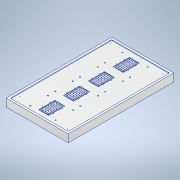
# Autodesk Inventor part: Tamale Assembly Plate 0p625in
Saved by Autodesk Inventor 2022 (Build 260153000, 153)
## iProperties
Created: 2021-07-29
Part Number: Tamale Assembly Plate 0p625in
Material: Aluminum 6061
Document SubType Name: Modeling
Designer: Caleb
Density: 2.7 g/cm^3
Appearance: Aluminum - Flat
Author: Caleb
Autodesk Inventor part; units mm, degrees
ref_plane "YZ Plane" through (0, 0, 0) normal (1, 0, 0) x (0, 1, 0)
ref_plane "XZ Plane" through (0, 0, 0) normal (0, 1, 0) x (-1, 0, 0)
ref_plane "XY Plane" through (0, 0, 0) normal (0, 0, 1) x (1, 0, 0)
sketch "Sketch1" plane through (0, 0, 0) normal (0, 1, 0) x (-1, 0, 0)
  line L0 (-63.5, -107.95) -> (63.5, -107.95)
  line L1 (63.5, -107.95) -> (63.5, 107.95)
  line L2 (63.5, 107.95) -> (-63.5, 107.95)
  line L3 (-63.5, 107.95) -> (-63.5, -107.95)
  line L4 (-63.5, -107.95) -> (63.5, 107.95) construction
  line L5 (63.5, -107.95) -> (-63.5, 107.95) construction
  point P0 (0, 0)
  dimension "d0" = 127
  dimension "d1" = 215.9
  constraints: 12 end point, 2 midpoint, 2 parallel, 1 horizontal, 1 perpendicular
  measures "d0" distance of L2.end L1.end
  measures "d1" distance of L0.end L1.end
extrude "Extrusion1" add sketch "Sketch1" along normal blind 15.875
sketch "Sketch2" plane through (0, 15.875, 0) normal (0, 1, 0) x (1, 0, 0)
  line L0 (57.15, 103.6) -> (-57.15, 103.6)
  line L1 (-59.15, 101.6) -> (-59.15, -101.6)
  line L2 (-57.15, -103.6) -> (57.15, -103.6)
  line L3 (59.15, -101.6) -> (59.15, 101.6)
  line L4 (59.15, 103.6) -> (-59.15, -103.6) construction
  line L5 (-59.15, 103.6) -> (59.15, -103.6) construction
  line L6 (-63.5, -107.95) -> (63.5, -107.95) projected
  line L7 (-63.5, 107.95) -> (-63.5, -107.95) projected
  line L8 (63.5, 107.95) -> (-63.5, 107.95) projected
  line L9 (63.5, -107.95) -> (63.5, 107.95) projected
  arc A0 (-59.15, -101.6) -> (-57.15, -103.6) centre (-57.15, -101.6) ccw
  arc A1 (57.15, -103.6) -> (59.15, -101.6) centre (57.15, -101.6) ccw
  arc A2 (59.15, 101.6) -> (57.15, 103.6) centre (57.15, 101.6) ccw
  arc A3 (-57.15, 103.6) -> (-59.15, 101.6) centre (-57.15, 101.6) ccw
  point P0 (0, 0)
  dimension "d4" = 4.35
  dimension "d5" = 4.35
  dimension "d6" = 4.35
  dimension "d77" = 2
  constraints: 12 end point, 8 point on circle, 8 point on line, 8 tangent, 4 centre point, 3 equal radius, 2 midpoint, 2 parallel, 1 horizontal, 1 perpendicular
  measures "d4" distance between parallel lines of L2 L6
  measures "d5" distance between parallel lines of L0 L8
  measures "d6" distance between parallel lines of L7 L1
  measures "d77" radius of A0
extrude "Extrusion2" cut sketch "Sketch2" against normal blind 1.6 contours A2 L3 A1 L2 A0 L1 A3 L0
sketch "Sketch3" plane through (0, 14.275, 0) normal (0, 1, 0) x (1, 0, 0)
  line L0 (-59.15, -101.6) -> (-59.15, 101.6) projected
  line L1 (57.15, -103.6) -> (-57.15, -103.6) projected
  point P0 (0, 0)
  point P1 (-26.75, -95.25)
  point P2 (-26.75, -59.15)
  point P3 (24.75, -95.25)
  point P4 (24.75, -59.15)
  point P5 (-57.15, -101.6)
  point P6 (-57.15, 101.6)
  point P7 (57.15, -101.6)
  point P8 (-26.75, -44.45)
  point P9 (24.75, -44.45)
  point P10 (24.75, -8.35)
  point P11 (-26.75, -8.35)
  point P12 (-26.75, 6.35)
  point P13 (24.75, 6.35)
  point P14 (24.75, 42.45)
  point P15 (-26.75, 42.45)
  point P16 (-26.75, 57.15)
  point P17 (24.75, 57.15)
  point P18 (24.75, 93.25)
  point P19 (-26.75, 93.25)
  point P20 (-59.15, 101.6)
  point P21 (-57.15, -103.6)
  dimension "d9" = 32.4
  dimension "d10" = 8.35
  dimension "d11" = 36.1
  dimension "d12" = 51.5
  dimension "d15" = 50.8
  constraints: 14 vertical alignment, 2 horizontal alignment, 2 other
  measures "d11" distance of point (-26.75, -59.15) point (-26.75, -95.25)
  measures "d12" distance of point (24.75, -59.15) point (-26.75, -59.15)
  measures "d15" distance of point (-26.75, -95.25) point (-26.75, -44.45)
hole "Hole1" at (-26.75, 14.275, 95.25) at (-26.75, 14.275, 59.15) at (24.75, 14.275, 95.25) at (24.75, 14.275, 59.15) at (-26.75, 14.275, 44.45) at (24.75, 14.275, 44.45) at (24.75, 14.275, 8.35) at (-26.75, 14.275, 8.35) at (-26.75, 14.275, -6.35) at (24.75, 14.275, -6.35) at (24.75, 14.275, -42.45) at (-26.75, 14.275, -42.45) at (-26.75, 14.275, -57.15) at (24.75, 14.275, -57.15) at (24.75, 14.275, -93.25) at (-26.75, 14.275, -93.25) direction (0, -1, 0) diameter 2.5 end through all
sketch "Sketch4" plane through (0, 14.275, 0) normal (0, 1, 0) x (1, 0, 0)
  line L0 (-59.15, -101.6) -> (-59.15, 101.6) projected
  line L1 (57.15, -103.6) -> (-57.15, -103.6) projected
  line L2 (59.15, 101.6) -> (59.15, -101.6) projected
  line L3 (-57.15, 103.6) -> (57.15, 103.6) projected
  point P0 (0, 0)
  point P1 (-54.15, -88.9)
  point P2 (-57.15, -101.6)
  point P3 (-57.15, 101.6)
  point P4 (57.15, -101.6)
  point P5 (52.155, -98.61)
  point P6 (52.155, 96.6)
  point P7 (-54.135, 96.6)
  point P8 (57.15, 101.6)
  point P9 (-12.765, -85.2)
  point P10 (-12.765, -69.2)
  point P11 (10.766, -85.2)
  point P12 (10.766, -69.2)
  point P13 (-12.765, -34.4)
  point P14 (-12.765, -18.4)
  point P15 (10.766, -18.4)
  point P16 (10.766, -34.4)
  point P17 (-12.765, 16.4)
  point P18 (-12.765, 32.4)
  point P19 (10.766, 32.4)
  point P20 (10.766, 16.4)
  point P21 (-12.765, 67.2)
  point P22 (-12.765, 83.2)
  point P23 (10.766, 83.2)
  point P24 (10.766, 67.2)
  point P25 (-59.15, 101.6)
  point P26 (-57.15, -103.6)
  point P27 (59.15, -101.6)
  point P28 (57.15, 103.6)
  dimension "d35" = 46.385
  dimension "d36" = 18.4
  dimension "d37" = 16
  dimension "d38" = 23.531
  dimension "d41" = 50.8
  dimension "d98" = 3.7
  dimension "d99" = 41.385
  dimension "d100" = 13.41
  dimension "d101" = 64.92
  dimension "d102" = 181.8
  dimension "d103" = 41.37
  dimension "d104" = 181.8
  dimension "d105" = 64.92
  constraints: 14 vertical alignment, 2 horizontal alignment, 4 other
  measures "d37" distance of point (-12.765, -69.2) point (-12.765, -85.2)
  measures "d38" distance of point (10.766, -85.2) point (-12.765, -85.2)
  measures "d41" distance of point (-12.765, -85.2) point (-12.765, -34.4)
  measures "d98" vertical distance of point (-54.15, -88.9) point (-12.765, -85.2)
  measures "d99" horizontal distance of point (-12.765, -85.2) point (-54.15, -88.9)
  measures "d100" vertical distance of point (52.155, -98.61) point (-12.765, -85.2)
  measures "d101" horizontal distance of point (52.155, -98.61) point (-12.765, -85.2)
  measures "d102" vertical distance of point (-12.765, -85.2) point (-54.135, 96.6)
  measures "d103" horizontal distance of point (-12.765, -85.2) point (-54.135, 96.6)
  measures "d104" vertical distance of point (52.155, 96.6) point (-12.765, -85.2)
  measures "d105" horizontal distance of point (52.155, 96.6) point (-12.765, -85.2)
hole "Hole2" at (-54.15, 14.275, 88.9) at (52.155, 14.275, 98.61) at (52.155, 14.275, -96.6) at (-54.135, 14.275, -96.6) at (-12.765, 14.275, 85.2) at (-12.765, 14.275, 69.2) at (10.766, 14.275, 85.2) at (10.766, 14.275, 69.2) at (-12.765, 14.275, 34.4) at (-12.765, 14.275, 18.4) at (10.766, 14.275, 18.4) at (10.766, 14.275, 34.4) at (-12.765, 14.275, -16.4) at (-12.765, 14.275, -32.4) at (10.766, 14.275, -32.4) at (10.766, 14.275, -16.4) at (-12.765, 14.275, -67.2) at (-12.765, 14.275, -83.2) at (10.766, 14.275, -83.2) at (10.766, 14.275, -67.2) direction (0, -1, 0) diameter 1.0211 end through all thread size "00-96 NS" class "2B" standard "ANSI Unified Screw Threads"
sketch "Sketch5" plane through (0, 14.275, 0) normal (0, 1, 0) x (1, 0, 0)
  line L0 (57.15, -103.6) -> (-57.15, -103.6) projected
  line L1 (-59.15, -101.6) -> (-59.15, 101.6) projected
  point P0 (0, 0)
  point P1 (-7.35, -89.9)
  point P2 (57.15, -101.6)
  point P3 (-57.15, -101.6)
  point P4 (-57.15, 101.6)
  point P5 (-7.35, -86.725)
  point P6 (-7.35, -83.55)
  point P7 (-7.35, -80.375)
  point P8 (-7.35, -77.2)
  point P9 (-7.35, -74.025)
  point P10 (-7.35, -70.85)
  point P11 (-7.35, -67.675)
  point P12 (-7.35, -64.5)
  point P13 (-4.175, -89.9)
  point P14 (-4.175, -86.725)
  point P15 (-4.175, -83.55)
  point P16 (-4.175, -80.375)
  point P17 (-4.175, -77.2)
  point P18 (-4.175, -74.025)
  point P19 (-4.175, -70.85)
  point P20 (-4.175, -67.675)
  point P21 (-4.175, -64.5)
  point P22 (-1, -89.9)
  point P23 (-1, -86.725)
  point P24 (-1, -83.55)
  point P25 (-1, -80.375)
  point P26 (-1, -77.2)
  point P27 (-1, -74.025)
  point P28 (-1, -70.85)
  point P29 (-1, -67.675)
  point P30 (-1, -64.5)
  point P31 (2.175, -89.9)
  point P32 (2.175, -86.725)
  point P33 (2.175, -83.55)
  point P34 (2.175, -80.375)
  point P35 (2.175, -77.2)
  point P36 (2.175, -74.025)
  point P37 (2.175, -70.85)
  point P38 (2.175, -67.675)
  point P39 (2.175, -64.5)
  point P40 (5.35, -89.9)
  point P41 (5.35, -86.725)
  point P42 (5.35, -83.55)
  point P43 (5.35, -80.375)
  point P44 (5.35, -77.2)
  point P45 (5.35, -74.025)
  point P46 (5.35, -70.85)
  point P47 (5.35, -67.675)
  point P48 (5.35, -64.5)
  point P49 (5.35, -13.7)
  point P50 (5.35, -16.875)
  point P51 (5.35, -20.05)
  point P52 (5.35, -23.225)
  point P53 (5.35, -26.4)
  point P54 (5.35, -29.575)
  point P55 (5.35, -32.75)
  point P56 (5.35, -35.925)
  point P57 (5.35, -39.1)
  point P58 (2.175, -13.7)
  point P59 (2.175, -16.875)
  point P60 (2.175, -20.05)
  point P61 (2.175, -23.225)
  point P62 (2.175, -26.4)
  point P63 (2.175, -29.575)
  point P64 (2.175, -32.75)
  point P65 (2.175, -35.925)
  point P66 (2.175, -39.1)
  point P67 (-1, -13.7)
  point P68 (-1, -16.875)
  point P69 (-1, -20.05)
  point P70 (-1, -23.225)
  point P71 (-1, -26.4)
  point P72 (-1, -29.575)
  point P73 (-1, -32.75)
  point P74 (-1, -35.925)
  point P75 (-1, -39.1)
  point P76 (-4.175, -13.7)
  point P77 (-4.175, -16.875)
  point P78 (-4.175, -20.05)
  point P79 (-4.175, -23.225)
  point P80 (-4.175, -26.4)
  point P81 (-4.175, -29.575)
  point P82 (-4.175, -32.75)
  point P83 (-4.175, -35.925)
  point P84 (-4.175, -39.1)
  point P85 (-7.35, -13.7)
  point P86 (-7.35, -16.875)
  point P87 (-7.35, -20.05)
  point P88 (-7.35, -23.225)
  point P89 (-7.35, -26.4)
  point P90 (-7.35, -29.575)
  point P91 (-7.35, -32.75)
  point P92 (-7.35, -35.925)
  point P93 (-7.35, -39.1)
  point P94 (5.35, 37.1)
  point P95 (5.35, 33.925)
  point P96 (5.35, 30.75)
  point P97 (5.35, 27.575)
  point P98 (5.35, 24.4)
  point P99 (5.35, 21.225)
  point P100 (5.35, 18.05)
  point P101 (5.35, 14.875)
  point P102 (5.35, 11.7)
  point P103 (2.175, 37.1)
  point P104 (2.175, 33.925)
  point P105 (2.175, 30.75)
  point P106 (2.175, 27.575)
  point P107 (2.175, 24.4)
  point P108 (2.175, 21.225)
  point P109 (2.175, 18.05)
  point P110 (2.175, 14.875)
  point P111 (2.175, 11.7)
  point P112 (-1, 37.1)
  point P113 (-1, 33.925)
  point P114 (-1, 30.75)
  point P115 (-1, 27.575)
  point P116 (-1, 24.4)
  point P117 (-1, 21.225)
  point P118 (-1, 18.05)
  point P119 (-1, 14.875)
  point P120 (-1, 11.7)
  point P121 (-4.175, 37.1)
  point P122 (-4.175, 33.925)
  point P123 (-4.175, 30.75)
  point P124 (-4.175, 27.575)
  point P125 (-4.175, 24.4)
  point P126 (-4.175, 21.225)
  point P127 (-4.175, 18.05)
  point P128 (-4.175, 14.875)
  point P129 (-4.175, 11.7)
  point P130 (-7.35, 37.1)
  point P131 (-7.35, 33.925)
  point P132 (-7.35, 30.75)
  point P133 (-7.35, 27.575)
  point P134 (-7.35, 24.4)
  point P135 (-7.35, 21.225)
  point P136 (-7.35, 18.05)
  point P137 (-7.35, 14.875)
  point P138 (-7.35, 11.7)
  point P139 (5.35, 87.9)
  point P140 (5.35, 84.725)
  point P141 (5.35, 81.55)
  point P142 (5.35, 78.375)
  point P143 (5.35, 75.2)
  point P144 (5.35, 72.025)
  point P145 (5.35, 68.85)
  point P146 (5.35, 65.675)
  point P147 (5.35, 62.5)
  point P148 (2.175, 87.9)
  point P149 (2.175, 84.725)
  point P150 (2.175, 81.55)
  point P151 (2.175, 78.375)
  point P152 (2.175, 75.2)
  point P153 (2.175, 72.025)
  point P154 (2.175, 68.85)
  point P155 (2.175, 65.675)
  point P156 (2.175, 62.5)
  point P157 (-1, 87.9)
  point P158 (-1, 84.725)
  point P159 (-1, 81.55)
  point P160 (-1, 78.375)
  point P161 (-1, 75.2)
  point P162 (-1, 72.025)
  point P163 (-1, 68.85)
  point P164 (-1, 65.675)
  point P165 (-1, 62.5)
  point P166 (-4.175, 87.9)
  point P167 (-4.175, 84.725)
  point P168 (-4.175, 81.55)
  point P169 (-4.175, 78.375)
  point P170 (-4.175, 75.2)
  point P171 (-4.175, 72.025)
  point P172 (-4.175, 68.85)
  point P173 (-4.175, 65.675)
  point P174 (-4.175, 62.5)
  point P175 (-7.35, 87.9)
  point P176 (-7.35, 84.725)
  point P177 (-7.35, 81.55)
  point P178 (-7.35, 78.375)
  point P179 (-7.35, 75.2)
  point P180 (-7.35, 72.025)
  point P181 (-7.35, 68.85)
  point P182 (-7.35, 65.675)
  point P183 (-7.35, 62.5)
  point P184 (-57.15, -103.6)
  point P185 (-59.15, 101.6)
  dimension "d53" = 13.7
  dimension "d54" = 51.8
  dimension "d57" = 3.175
  dimension "d60" = 3.175
  dimension "d65" = 50.8
  constraints: 143 vertical alignment, 36 horizontal alignment, 2 other
  measures "d57" distance of point (-7.35, -89.9) point (-7.35, -86.725)
  measures "d60" distance of point (-7.35, -89.9) point (-4.175, -89.9)
  measures "d65" distance of point (5.35, -64.5) point (5.35, -13.7)
hole "Hole3" at (-7.35, 14.275, 89.9) at (-7.35, 14.275, 86.725) at (-7.35, 14.275, 83.55) at (-7.35, 14.275, 80.375) at (-7.35, 14.275, 77.2) at (-7.35, 14.275, 74.025) at (-7.35, 14.275, 70.85) at (-7.35, 14.275, 67.675) at (-7.35, 14.275, 64.5) at (-4.175, 14.275, 89.9) at (-4.175, 14.275, 86.725) at (-4.175, 14.275, 83.55) at (-4.175, 14.275, 80.375) at (-4.175, 14.275, 77.2) at (-4.175, 14.275, 74.025) at (-4.175, 14.275, 70.85) at (-4.175, 14.275, 67.675) at (-4.175, 14.275, 64.5) at (-1, 14.275, 89.9) at (-1, 14.275, 86.725) at (-1, 14.275, 83.55) at (-1, 14.275, 80.375) at (-1, 14.275, 77.2) at (-1, 14.275, 74.025) at (-1, 14.275, 70.85) at (-1, 14.275, 67.675) at (-1, 14.275, 64.5) at (2.175, 14.275, 89.9) at (2.175, 14.275, 86.725) at (2.175, 14.275, 83.55) at (2.175, 14.275, 80.375) at (2.175, 14.275, 77.2) at (2.175, 14.275, 74.025) at (2.175, 14.275, 70.85) at (2.175, 14.275, 67.675) at (2.175, 14.275, 64.5) at (5.35, 14.275, 89.9) at (5.35, 14.275, 86.725) at (5.35, 14.275, 83.55) at (5.35, 14.275, 80.375) at (5.35, 14.275, 77.2) at (5.35, 14.275, 74.025) at (5.35, 14.275, 70.85) at (5.35, 14.275, 67.675) at (5.35, 14.275, 64.5) at (5.35, 14.275, 13.7) at (5.35, 14.275, 16.875) at (5.35, 14.275, 20.05) at (5.35, 14.275, 23.225) at (5.35, 14.275, 26.4) direction (0, -1, 0) diameter 1.6 end through all and at (5.35, 14.275, 29.575) (5.35, 14.275, 32.75) (5.35, 14.275, 35.925) (5.35, 14.275, 39.1) (2.175, 14.275, 13.7) (2.175, 14.275, 16.875) (2.175, 14.275, 20.05) (2.175, 14.275, 23.225) (2.175, 14.275, 26.4) (2.175, 14.275, 29.575) (2.175, 14.275, 32.75) (2.175, 14.275, 35.925) (2.175, 14.275, 39.1) (-1, 14.275, 13.7) (-1, 14.275, 16.875) (-1, 14.275, 20.05) (-1, 14.275, 23.225) (-1, 14.275, 26.4) (-1, 14.275, 29.575) (-1, 14.275, 32.75) (-1, 14.275, 35.925) (-1, 14.275, 39.1) (-4.175, 14.275, 13.7) (-4.175, 14.275, 16.875) (-4.175, 14.275, 20.05) (-4.175, 14.275, 23.225) (-4.175, 14.275, 26.4) (-4.175, 14.275, 29.575) (-4.175, 14.275, 32.75) (-4.175, 14.275, 35.925) (-4.175, 14.275, 39.1) (-7.35, 14.275, 13.7) (-7.35, 14.275, 16.875) (-7.35, 14.275, 20.05) (-7.35, 14.275, 23.225) (-7.35, 14.275, 26.4) (-7.35, 14.275, 29.575) (-7.35, 14.275, 32.75) (-7.35, 14.275, 35.925) (-7.35, 14.275, 39.1) (5.35, 14.275, -37.1) (5.35, 14.275, -33.925) (5.35, 14.275, -30.75) (5.35, 14.275, -27.575) (5.35, 14.275, -24.4) (5.35, 14.275, -21.225) (5.35, 14.275, -18.05) (5.35, 14.275, -14.875) (5.35, 14.275, -11.7) (2.175, 14.275, -37.1) (2.175, 14.275, -33.925) (2.175, 14.275, -30.75) (2.175, 14.275, -27.575) (2.175, 14.275, -24.4) (2.175, 14.275, -21.225) (2.175, 14.275, -18.05) (2.175, 14.275, -14.875) (2.175, 14.275, -11.7) (-1, 14.275, -37.1) (-1, 14.275, -33.925) (-1, 14.275, -30.75) (-1, 14.275, -27.575) (-1, 14.275, -24.4) (-1, 14.275, -21.225) (-1, 14.275, -18.05) (-1, 14.275, -14.875) (-1, 14.275, -11.7) (-4.175, 14.275, -37.1) (-4.175, 14.275, -33.925) (-4.175, 14.275, -30.75) (-4.175, 14.275, -27.575) (-4.175, 14.275, -24.4) (-4.175, 14.275, -21.225) (-4.175, 14.275, -18.05) (-4.175, 14.275, -14.875) (-4.175, 14.275, -11.7) (-7.35, 14.275, -37.1) (-7.35, 14.275, -33.925) (-7.35, 14.275, -30.75) (-7.35, 14.275, -27.575) (-7.35, 14.275, -24.4) (-7.35, 14.275, -21.225) (-7.35, 14.275, -18.05) (-7.35, 14.275, -14.875) (-7.35, 14.275, -11.7) (5.35, 14.275, -87.9) (5.35, 14.275, -84.725) (5.35, 14.275, -81.55) (5.35, 14.275, -78.375) (5.35, 14.275, -75.2) (5.35, 14.275, -72.025) (5.35, 14.275, -68.85) (5.35, 14.275, -65.675) (5.35, 14.275, -62.5) (2.175, 14.275, -87.9) (2.175, 14.275, -84.725) (2.175, 14.275, -81.55) (2.175, 14.275, -78.375) (2.175, 14.275, -75.2) (2.175, 14.275, -72.025) (2.175, 14.275, -68.85) (2.175, 14.275, -65.675) (2.175, 14.275, -62.5) (-1, 14.275, -87.9) (-1, 14.275, -84.725) (-1, 14.275, -81.55) (-1, 14.275, -78.375) (-1, 14.275, -75.2) (-1, 14.275, -72.025) (-1, 14.275, -68.85) (-1, 14.275, -65.675) (-1, 14.275, -62.5) (-4.175, 14.275, -87.9) (-4.175, 14.275, -84.725) (-4.175, 14.275, -81.55) (-4.175, 14.275, -78.375) (-4.175, 14.275, -75.2) (-4.175, 14.275, -72.025) (-4.175, 14.275, -68.85) (-4.175, 14.275, -65.675) (-4.175, 14.275, -62.5) (-7.35, 14.275, -87.9) (-7.35, 14.275, -84.725) (-7.35, 14.275, -81.55) (-7.35, 14.275, -78.375) (-7.35, 14.275, -75.2) (-7.35, 14.275, -72.025) (-7.35, 14.275, -68.85) (-7.35, 14.275, -65.675) (-7.35, 14.275, -62.5)
sketch "Sketch6" plane through (0, 14.275, 0) normal (0, 1, 0) x (1, 0, 0)
  line L0 (5.95, -62.4) -> (-7.95, -62.4)
  line L1 (-9.45, -63.9) -> (-9.45, -90.5)
  line L2 (-7.95, -92) -> (5.95, -92)
  line L3 (7.45, -90.5) -> (7.45, -63.9)
  line L4 (7.982, -60.368) -> (-9.982, -60.368)
  line L5 (-11.482, -61.868) -> (-11.482, -92.532)
  line L6 (-9.982, -94.032) -> (7.982, -94.032)
  line L7 (9.482, -92.532) -> (9.482, -61.868)
  circle A0 centre (-7.35, -64.5) radius 0.8 projected
  circle A1 centre (-7.35, -89.9) radius 0.8 projected
  circle A2 centre (5.35, -89.9) radius 0.8 projected
  arc A3 (-9.45, -90.5) -> (-7.95, -92) centre (-7.95, -90.5) ccw
  arc A4 (-11.482, -92.532) -> (-9.982, -94.032) centre (-9.982, -92.532) ccw
  arc A5 (-9.982, -60.368) -> (-11.482, -61.868) centre (-9.982, -61.868) ccw
  arc A6 (-7.95, -62.4) -> (-9.45, -63.9) centre (-7.95, -63.9) ccw
  arc A7 (7.45, -63.9) -> (5.95, -62.4) centre (5.95, -63.9) ccw
  arc A8 (9.482, -61.868) -> (7.982, -60.368) centre (7.982, -61.868) ccw
  arc A9 (7.982, -94.032) -> (9.482, -92.532) centre (7.982, -92.532) ccw
  arc A10 (5.95, -92) -> (7.45, -90.5) centre (5.95, -90.5) ccw
  line L8 (-7.95, -41.2) -> (5.95, -41.2)
  line L9 (-9.982, -43.232) -> (7.982, -43.232)
  arc A11 (5.95, -41.2) -> (7.45, -39.7) centre (5.95, -39.7) ccw
  arc A12 (7.982, -43.232) -> (9.482, -41.732) centre (7.982, -41.732) ccw
  arc A13 (-9.45, -39.7) -> (-7.95, -41.2) centre (-7.95, -39.7) ccw
  arc A14 (-11.482, -41.732) -> (-9.982, -43.232) centre (-9.982, -41.732) ccw
  line L10 (5.95, -11.6) -> (-7.95, -11.6)
  line L11 (-9.45, -13.1) -> (-9.45, -39.7)
  line L12 (7.45, -39.7) -> (7.45, -13.1)
  line L13 (7.982, -9.568) -> (-9.982, -9.568)
  line L14 (-11.482, -11.068) -> (-11.482, -41.732)
  line L15 (9.482, -41.732) -> (9.482, -11.068)
  arc A15 (-7.95, -11.6) -> (-9.45, -13.1) centre (-7.95, -13.1) ccw
  arc A16 (-9.982, -9.568) -> (-11.482, -11.068) centre (-9.982, -11.068) ccw
  arc A17 (9.482, -11.068) -> (7.982, -9.568) centre (7.982, -11.068) ccw
  arc A18 (7.45, -13.1) -> (5.95, -11.6) centre (5.95, -13.1) ccw
  line L16 (-7.95, 9.6) -> (5.95, 9.6)
  line L17 (-9.982, 7.568) -> (7.982, 7.568)
  arc A19 (5.95, 9.6) -> (7.45, 11.1) centre (5.95, 11.1) ccw
  arc A20 (7.982, 7.568) -> (9.482, 9.068) centre (7.982, 9.068) ccw
  arc A21 (-9.45, 11.1) -> (-7.95, 9.6) centre (-7.95, 11.1) ccw
  arc A22 (-11.482, 9.068) -> (-9.982, 7.568) centre (-9.982, 9.068) ccw
  line L18 (5.95, 39.2) -> (-7.95, 39.2)
  line L19 (-9.45, 37.7) -> (-9.45, 11.1)
  line L20 (7.45, 11.1) -> (7.45, 37.7)
  line L21 (7.982, 41.232) -> (-9.982, 41.232)
  line L22 (-11.482, 39.732) -> (-11.482, 9.068)
  line L23 (9.482, 9.068) -> (9.482, 39.732)
  arc A23 (-7.95, 39.2) -> (-9.45, 37.7) centre (-7.95, 37.7) ccw
  arc A24 (-9.982, 41.232) -> (-11.482, 39.732) centre (-9.982, 39.732) ccw
  arc A25 (9.482, 39.732) -> (7.982, 41.232) centre (7.982, 39.732) ccw
  arc A26 (7.45, 37.7) -> (5.95, 39.2) centre (5.95, 37.7) ccw
  line L24 (-7.95, 60.4) -> (5.95, 60.4)
  line L25 (-9.982, 58.368) -> (7.982, 58.368)
  arc A27 (5.95, 60.4) -> (7.45, 61.9) centre (5.95, 61.9) ccw
  arc A28 (7.982, 58.368) -> (9.482, 59.868) centre (7.982, 59.868) ccw
  arc A29 (-9.45, 61.9) -> (-7.95, 60.4) centre (-7.95, 61.9) ccw
  arc A30 (-11.482, 59.868) -> (-9.982, 58.368) centre (-9.982, 59.868) ccw
  line L26 (5.95, 90) -> (-7.95, 90)
  line L27 (-9.45, 88.5) -> (-9.45, 61.9)
  line L28 (7.45, 61.9) -> (7.45, 88.5)
  line L29 (7.982, 92.032) -> (-9.982, 92.032)
  line L30 (-11.482, 90.532) -> (-11.482, 59.868)
  line L31 (9.482, 59.868) -> (9.482, 90.532)
  arc A31 (-7.95, 90) -> (-9.45, 88.5) centre (-7.95, 88.5) ccw
  arc A32 (-9.982, 92.032) -> (-11.482, 90.532) centre (-9.982, 90.532) ccw
  arc A33 (9.482, 90.532) -> (7.982, 92.032) centre (7.982, 90.532) ccw
  arc A34 (7.45, 88.5) -> (5.95, 90) centre (5.95, 88.5) ccw
  point P0 (0, 0)
  dimension "d79" = 2.1
  dimension "d80" = 2.1
  dimension "d81" = 2.1
  dimension "d82" = 2.1
  dimension "d83" = 2.032
  dimension "d84" = 2.032
  dimension "d85" = 2.032
  dimension "d86" = 2.032
  dimension "d87" = 1.5
  dimension "d88" = 1.5
  dimension "d91" = 50.8
  constraints: 64 end point, 64 point on circle, 32 centre point, 16 tangent, 6 equal radius, 4 parallel, 2 horizontal, 2 perpendicular, 1 collinear, 1 vertical, 119 other
  measures "d79" distance from line of A1.centre L2
  measures "d80" distance from line of L0 A0.centre
  measures "d81" distance from line of L1 A0.centre
  measures "d82" distance from line of L3 A2.centre
  measures "d83" distance between parallel lines of L6 L2
  measures "d84" distance between parallel lines of L1 L5
  measures "d85" distance between parallel lines of L7 L3
  measures "d86" distance between parallel lines of L0 L4
  measures "d87" radius of A3
  measures "d88" radius of A4
  measures "d91" distance of L2.start L8.start
extrude "Extrusion3" cut sketch "Sketch6" against normal blind 1.143 contours A8 L7 A9 L6 A4 L5 A5 L4 | A14 L14 A16 L13 A17 L15 A12 L9 | A22 L22 A24 L21 A25 L23 A20 L17 | A30 L30 A32 L29 A33 L31 A28 L25
body "Solid1"
